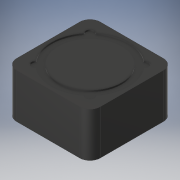
# Autodesk Inventor part: coil
Saved by Autodesk Inventor 2019 (Build 230136000, 136)
## iProperties
Created: 2020-02-18
Part Number: coil
Material: Generic
Document SubType Name: Modeling
Designer: close
Density: 1 g/cm^3
Appearance: Smooth - Black
Author: close
Autodesk Inventor part; units mm, degrees
ref_plane "YZ Plane" through (0, 0, 0) normal (1, 0, 0) x (0, 1, 0)
ref_plane "XZ Plane" through (0, 0, 0) normal (0, 1, 0) x (-1, 0, 0)
ref_plane "XY Plane" through (0, 0, 0) normal (0, 0, 1) x (1, 0, 0)
sketch "Sketch1" plane through (0, 0, 0) normal (0, 1, 0) x (-1, 0, 0)
  line L0 (1.5, 0) -> (10.75, 0)
  line L1 (12.25, -1.5) -> (12.25, -10.75)
  line L2 (10.75, -12.25) -> (1.5, -12.25)
  line L3 (0, -10.75) -> (0, -1.5)
  arc A0 (12.25, -1.5) -> (10.75, 0) centre (10.75, -1.5) ccw
  arc A1 (10.75, -12.25) -> (12.25, -10.75) centre (10.75, -10.75) ccw
  arc A2 (0, -10.75) -> (1.5, -12.25) centre (1.5, -10.75) ccw
  arc A3 (1.5, 0) -> (0, -1.5) centre (1.5, -1.5) ccw
  point P0 (0, 0)
  point P1 (12.25, -12.25)
  point P2 (12.25, 0)
  dimension "d0" = 12.25
  dimension "d1" = 12.25
  dimension "d2" = 1.5
  constraints: 8 end point, 8 point on circle, 8 tangent, 6 point on line, 4 centre point, 3 equal radius, 2 parallel, 1 horizontal, 1 perpendicular
  measures "d0" distance of point (12.25, 0) point (12.25, -12.25)
  measures "d1" distance of point (0, 0) point (12.25, 0)
  measures "d2" radius of A0
extrude "Extrusion1" add sketch "Sketch1" along normal blind 6.5
sketch "Sketch2" plane through (0, 6.5, 0) normal (0, 1, 0) x (1, 0, 0)
  circle A0 centre (-6.125, 6.125) radius 5.625
  line L0 (-1.5, 12.25) -> (-10.75, 12.25) projected
  line L1 (-10.75, 0) -> (-1.5, 0) projected
  circle A1 centre (-6.125, 6.125) radius 4.625
  circle A2 centre (-10.1025, 2.1475) radius 0.625
  arc A3 (-12.25, 1.5) -> (-10.75, 0) centre (-10.75, 1.5) ccw construction
  line L2 (-6.125, 6.125) -> (-10.75, 1.5) construction
  line L3 (-12.25, 10.75) -> (-12.25, 1.5) construction
  circle A4 centre (-2.1475, 2.1475) radius 0.625
  circle A5 centre (-2.1475, 10.1025) radius 0.625
  circle A6 centre (-10.1025, 10.1025) radius 0.625
  point P0 (0, 0)
  dimension "d6" = 11.25
  dimension "d5" = 12.25
  dimension "d7" = 1
  dimension "d8" = 1.25
  dimension "d9" = 6.125
  dimension "d10" = 6.125
  dimension "d13" = 360
  constraints: 5 centre point, 2 end point, 1 coincident, 1 point on line, 12 other
  measures "d5" distance between parallel lines of L0 L1
  measures "d8" diameter of A2
  measures "d9" distance from line of L1 point (-6.125, 6.125)
  measures "d10" distance from line of L3 point (-6.125, 6.125)
extrude "Extrusion2" cut sketch "Sketch2" against normal blind 0.25
equation "\"d1\" = d0"
equation "\"d9\" = 0.5 * d5"
equation "\"d10\" = d9"
body "Solid1"
